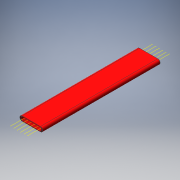
# Autodesk Inventor part: isolator_C
Saved by Autodesk Inventor 2016 SP1 (Build 200210100, 210)
## iProperties
Created: 2017-07-06
Part Number: isolator_C
Material: Типовые
Document SubType Name: Modeling
Designer: user
Density: 1 g/cm^3
Appearance: По умолчанию
Author: user
Autodesk Inventor part; units mm, degrees
ref_plane "YZ Plane" through (0, 0, 0) normal (1, 0, 0) x (0, 1, 0)
ref_plane "XZ Plane" through (0, 0, 0) normal (0, 1, 0) x (-1, 0, 0)
ref_plane "XY Plane" through (0, 0, 0) normal (0, 0, 1) x (1, 0, 0)
sketch "Эскиз1" plane through (0, 0, 0) normal (0, 1, 0) x (-1, 0, 0)
  line L0 (20.5571, -2.4) -> (-16.8429, -2.4)
  line L1 (-21.6429, -7.2) -> (-21.6429, -7.2)
  line L2 (-16.8429, -12) -> (20.5571, -12)
  line L3 (25.3571, -7.2) -> (25.3571, -7.2)
  arc A0 (25.3571, -7.2) -> (20.5571, -2.4) centre (20.5571, -7.2) ccw
  arc A1 (20.5571, -12) -> (25.3571, -7.2) centre (20.5571, -7.2) ccw
  arc A2 (-16.8429, -2.4) -> (-21.6429, -7.2) centre (-16.8429, -7.2) ccw
  arc A3 (-21.6429, -7.2) -> (-16.8429, -12) centre (-16.8429, -7.2) ccw
  line L4 (19.0571, -3.4) -> (-15.3429, -3.4)
  line L5 (-19.1429, -7.2) -> (-19.1429, -7.2)
  line L6 (-15.3429, -11) -> (19.0571, -11)
  line L7 (22.8571, -7.2) -> (22.8571, -7.2)
  arc A4 (22.8571, -7.2) -> (19.0571, -3.4) centre (19.0571, -7.2) ccw
  arc A5 (19.0571, -11) -> (22.8571, -7.2) centre (19.0571, -7.2) ccw
  arc A6 (-19.1429, -7.2) -> (-15.3429, -11) centre (-15.3429, -7.2) ccw
  arc A7 (-15.3429, -3.4) -> (-19.1429, -7.2) centre (-15.3429, -7.2) ccw
  point P0 (0, 0)
  point P1 (25.3571, -2.4)
  point P2 (-21.6429, -2.4)
  dimension "d0" = 47
  dimension "d1" = 9.6
  dimension "d2" = 4.8
  dimension "d3" = 1
  dimension "d4" = 1
  dimension "d5" = 2.5
  dimension "d6" = 2.5
  dimension "d7" = 3.8
  constraints: 16 end point, 16 point on circle, 16 tangent, 8 centre point, 6 equal radius, 4 parallel, 4 point on line, 2 horizontal, 2 perpendicular
  measures "d0" distance of point (-21.643, -2.4) point (25.357, -2.4)
  measures "d1" distance between parallel lines of L2 L0
  measures "d2" radius of A0
  measures "d3" distance between parallel lines of L4 L0
  measures "d4" distance between parallel lines of L2 L6
  measures "d5" distance from line of L3.end L7
  measures "d6" distance from line of L1.start L5
  measures "d7" radius of A4
extrude "Выдавливание1" add sketch "Эскиз1" along normal blind 240
ref_plane "РабПлоскость1" through (0, 250, 0) normal (0, 1, 0) x (1, 0, 0)
fillet "Сопряжение1" radius 0.5 24 edges at (-23.9513, 0, -3.8059) (-23.9513, 0, -10.5941) (-1.8571, 0, -12) (20.237, 0, -3.8059) (20.237, 0, -10.5941) (-1.8571, 0, -2.4) (18.0299, 0, -4.513) (18.0299, 0, -9.887) (-1.8571, 0, -11) (-21.7441, 0, -9.887) (-21.7441, 0, -4.513) (-1.8571, 0, -3.4) (-1.8571, 240, -11) (18.0299, 240, -4.513) (18.0299, 240, -9.887) (-1.8571, 240, -3.4) (-21.7441, 240, -9.887) (-21.7441, 240, -4.513) (-1.8571, 240, -2.4) (20.237, 240, -3.8059) (20.237, 240, -10.5941) (-1.8571, 240, -12) (-23.9513, 240, -3.8059) (-23.9513, 240, -10.5941)
ref_plane "РабПлоскость2" through (-19.0571, 0, -7.2) normal (0, 0, -1) x (0, 1, 0)
ref_plane "РабПлоскость4" through (-12.0571, 0, -7.2) normal (-1, 0, 0) x (0, 1, 0)
ref_plane "РабПлоскость3" through (-19.0571, 0, -7.2) normal (-1, 0, 0) x (0, 1, 0)
ref_plane "РабПлоскость5" through (-5.0571, 0, -7.2) normal (-1, 0, 0) x (0, 1, 0)
ref_plane "РабПлоскость6" through (1.9429, 0, -7.2) normal (-1, 0, 0) x (0, 1, 0)
ref_plane "РабПлоскость7" through (8.9429, 0, -7.2) normal (-1, 0, 0) x (0, 1, 0)
ref_plane "РабПлоскость8" through (15.9429, 0, -7.2) normal (-1, 0, 0) x (0, 1, 0)
